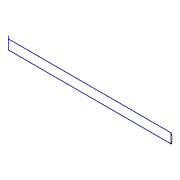
# Autodesk Inventor part: Heatsink Base
Saved by Autodesk Inventor 2020 (Build 240168000, 168)
## iProperties
Created: 2020-02-12
Part Number: Heatsink Base
Material: Generic
Document SubType Name: Modeling
Designer: ahamm
Density: 1 g/cm^3
Appearance: Default
Author: ahamm
Autodesk Inventor part; units mm, degrees
ref_plane "YZ Plane" through (0, 0, 0) normal (1, 0, 0) x (0, 1, 0)
ref_plane "XZ Plane" through (0, 0, 0) normal (0, 1, 0) x (-1, 0, 0)
ref_plane "XY Plane" through (0, 0, 0) normal (0, 0, 1) x (1, 0, 0)
sketch "Sketch1" plane through (0, 0, 0) normal (0, 0, 1) x (1, 0, 0)
  line L0 (-3.0081, 0) -> (-3.0081, -1.35)
  line L1 (-0.0086, -1.35) -> (-3.0081, -1.35) projected
  line L2 (81.9919, -1.35) -> (78.9914, -1.35) projected
  line L3 (78.9914, -1.35) -> (-0.0086, -1.35) projected
  line L4 (-3.0081, -1.35) -> (81.9919, -1.35)
  line L5 (81.9919, -1.35) -> (81.9919, -6.35)
  line L6 (81.9919, -6.35) -> (-3.0081, -6.35)
  line L7 (-3.0081, -6.35) -> (-3.0081, -1.35)
  line L8 (0, 12.6) -> (65.5305, 12.6) projected
  line L9 (0, 0) -> (0, 12.6) projected
  line L10 (0, 0) -> (3.1074, 0) projected
  line L11 (3.1074, 0) -> (3.1074, 4.1) projected
  line L12 (3.1074, 4.1) -> (39.418, 4.1) projected
  line L13 (39.418, 4.1) -> (39.418, 6.6) projected
  line L14 (39.418, 6.6) -> (54.418, 6.6) projected
  line L15 (54.418, 6.6) -> (54.418, 0) projected
  line L16 (54.418, 0) -> (60.3584, 0) projected
  line L17 (60.3584, 0) -> (60.3584, 1.0153) projected
  line L18 (60.3584, 1.0153) -> (65.5305, 1.0153) projected
  line L19 (65.5305, 1.0153) -> (65.5305, 12.6) projected
  dimension "d0" = 5
  constraints: 10 end point, 2 parallel, 1 horizontal, 1 perpendicular, 1 vertical, 2 other
  measures "d0" distance of L4.end L5.end
extrude "Extrusion1" add sketch "Sketch1" against normal blind 56.0375 contours L3 L2 L5 L6 L7 L1
fillet "Fillet1" radius 3 4 edges at (-3.0081, -3.85, 0) (-3.0081, -3.85, -56.0375) (81.9919, -3.85, 0) (81.9919, -3.85, -56.0375)
sketch "Sketch2" plane through (0, 0, 0) normal (0, 0, 1) x (1, 0, 0)
  line L0 (0, 12.6) -> (65.5305, 12.6) projected
  line L1 (0, 0) -> (0, 12.6) projected
  line L2 (0, 0) -> (3.1074, 0) projected
  line L3 (3.1074, 0) -> (3.1074, 4.1) projected
  line L4 (3.1074, 4.1) -> (39.418, 4.1) projected
  line L5 (39.418, 4.1) -> (39.418, 6.6) projected
  line L6 (39.418, 6.6) -> (54.418, 6.6) projected
  line L7 (54.418, 6.6) -> (54.418, 0) projected
  line L8 (54.418, 0) -> (60.3584, 0) projected
  line L9 (60.3584, 0) -> (60.3584, 1.0153) projected
  line L10 (60.3584, 1.0153) -> (65.5305, 1.0153) projected
  line L11 (65.5305, 1.0153) -> (65.5305, 12.6) projected
  line L12 (-0.0081, -1.35) -> (78.9919, -1.35) projected
  line L13 (3.1074, -1.35) -> (54.418, -1.35)
  line L14 (54.418, -1.35) -> (54.418, -4.7625)
  line L15 (54.418, -4.7625) -> (3.1074, -4.7625)
  line L16 (3.1074, -4.7625) -> (3.1074, -1.35)
  line L17 (60.3584, -1.5875) -> (89.6562, -1.5875)
  line L18 (89.6562, -1.5875) -> (89.6562, -4.7625)
  line L19 (89.6562, -4.7625) -> (60.3584, -4.7625)
  line L20 (60.3584, -4.7625) -> (60.3584, -1.5875)
  constraints: 16 end point, 4 parallel, 2 horizontal, 2 perpendicular, 2 point on line
extrude "Extrusion2" cut sketch "Sketch2" against normal blind 56.0375 contours L12 L14 L15 L16 | L17 L18 L19 L20
sketch "Sketch3" plane through (-3.0081, -6.35, -53.0375) normal (-1, 0, 0) x (0, 0, 1)
  line L0 (53.0375, 1.5875) -> (-3, 1.5875) projected
  line L1 (3.175, 1.5875) -> (46.9313, 1.5875)
  line L2 (46.9313, 1.5875) -> (46.9313, 6.35)
  line L3 (46.9313, 6.35) -> (3.175, 6.35)
  line L4 (3.175, 6.35) -> (3.175, 1.5875)
  point P0 (53.0375, 6.35)
  constraints: 8 end point, 2 parallel, 1 horizontal, 1 perpendicular, 1 point on line
extrude "Extrusion3" cut sketch "Sketch3" against normal blind 89.375
sketch "Sketch4" plane through (0, 0, 0) normal (0, 0, 1) x (1, 0, 0)
  line L0 (60.325, -1.5875) -> (82.55, -1.5875)
  line L1 (82.55, -1.5875) -> (82.55, 0)
  line L2 (82.55, 0) -> (60.325, 0)
  line L3 (60.325, 0) -> (60.325, -1.5875)
  point P0 (0, 0)
  constraints: 8 end point, 2 parallel, 1 horizontal, 1 perpendicular
extrude "Extrusion4" cut sketch "Sketch4" against normal blind 89.375
body "Solid1"
